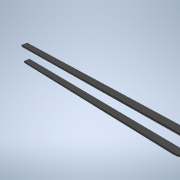
# Autodesk Inventor part: Belt_Z
Saved by Autodesk Inventor 2020 (Build 240168000, 168)
## iProperties
Created: 2020-03-07
Part Number: Belt_Z
Material: Rubber
Document SubType Name: Modeling
Designer: 10300812
Density: 0.93 g/cm^3
Appearance: Rubber - Black
Author: 10300812
Autodesk Inventor part; units mm, degrees
ref_plane "YZ Plane" through (0, 0, 0) normal (1, 0, 0) x (0, 1, 0)
ref_plane "XZ Plane" through (0, 0, 0) normal (0, 1, 0) x (-1, 0, 0)
ref_plane "XY Plane" through (0, 0, 0) normal (0, 0, 1) x (1, 0, 0)
sketch "Sketch1" plane through (0, 0, 0) normal (0, 0, 1) x (1, 0, 0)
  arc A0 (0, -6.05) -> (0, 6.05) centre (0, 0) ccw
  line L0 (0, -6.05) -> (-100, -6.05)
  line L1 (0, 6.05) -> (-100, 6.05)
  line L2 (-100, -7.55) -> (0, -7.55)
  arc A1 (0, -7.55) -> (0, 7.55) centre (0, 0) ccw
  line L3 (0, 7.55) -> (-100, 7.55)
  line L4 (-100, -7.55) -> (-100, -6.05)
  line L5 (-100, 6.05) -> (-100, 7.55)
  dimension "d0" = 12.1
  dimension "d1" = 100
  dimension "d2" = 1.5
  constraints: 12 end point, 4 point on circle, 2 centre point, 2 horizontal, 2 vertical alignment, 1 coincident, 1 collinear, 1 tangent, 1 vertical, 2 other
  measures "d0" diameter of A0
  measures "d1" distance of L0.start L0.end
  measures "d2" distance between parallel lines of L0 L2
extrude "Extrusion1" add sketch "Sketch1" along normal blind 5
body "Solid1"
